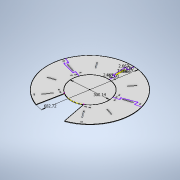
# Autodesk Inventor part: Ring Level 1 Full
Saved by Autodesk Inventor 2020 (Build 240168000, 168)
## iProperties
Created: 2020-03-10
Part Number: Ring Level 1 Full
Material: Generic
Document SubType Name: Sheet Metal
Designer: Daniel Wikman
Density: 1 g/cm^3
Sheet Metal Rule: Default_mm
Appearance: Default
Author: Daniel Wikman
Autodesk Inventor part; units mm, degrees
ref_plane "YZ Plane" through (0, 0, 0) normal (1, 0, 0) x (0, 1, 0)
ref_plane "XZ Plane" through (0, 0, 0) normal (0, 1, 0) x (-1, 0, 0)
sketch "Sketch1" plane through (0, 0, 0) normal (0, 1, 0) x (-1, 0, 0)
  circle A0 centre (0, 0) radius 341.36
  circle A1 centre (0, 0) radius 150.07
  dimension "d84" = 300.14
  dimension "d85" = 682.72
  constraints: 2 centre point, 1 coincident
  measures "d84" diameter of A1
  measures "d85" diameter of A0
extrude "Extrusion3" add sketch "Sketch1" along normal blind 6 contours A0 | A1
sketch "Sketch2" plane through (0, 6, 0) normal (0, 1, 0) x (1, 0, 0)
  circle A0 centre (0, 0) radius 245.715 construction
  line L0 (245.7148, 0.3131) -> (341.6521, -0.0088)
  line L1 (-0.6289, 279.0483) -> (-0.0524, 279.0483)
  line L2 (3.25, 279.0483) -> (3.25, 212.3817)
  line L3 (0.5377, 212.3817) -> (-0.051, 212.3817)
  line L4 (-3.25, 212.3817) -> (-3.25, 279.0483)
  arc A1 (-3.25, 212.3817) -> (-1.9167, 211.0483) centre (-1.9167, 212.3817) ccw
  arc A2 (1.9167, 211.0483) -> (3.25, 212.3817) centre (1.9167, 212.3817) ccw
  arc A3 (-1.9167, 280.3817) -> (-3.25, 279.0483) centre (-1.9167, 279.0483) ccw
  arc A4 (3.25, 279.0483) -> (1.9167, 280.3817) centre (1.9167, 279.0483) ccw
  line L5 (-1.9167, 280.3817) -> (1.9167, 280.3817)
  line L6 (-1.9167, 211.0483) -> (1.9167, 211.0483)
  line L7 (0, 0) -> (0, 212.3817)
  line L8 (0, 280.3817) -> (0, 341.36)
  line L9 (0, 211.0483) -> (0, 245.715) construction
  line L10 (0, 280.3817) -> (0, 245.715) construction
  arc A5 (-157.4948, 221.8428) -> (-159.3572, 222.1378) centre (-158.5735, 221.0591) ccw
  line L11 (-162.4585, 219.8846) -> (-159.3572, 222.1378)
  arc A6 (-162.4585, 219.8846) -> (-162.7534, 218.0222) centre (-161.6748, 218.8059) ccw
  line L12 (-160.9079, 221.0112) -> (-144.3647, 198.2416) construction
  line L13 (-160.633, 219.5628) -> (-160.1666, 219.9017)
  line L14 (-157.4948, 221.8428) -> (-125.976, 178.4609)
  line L15 (-131.2346, 174.6403) -> (-162.7534, 218.0222)
  line L16 (-127.8216, 175.4719) -> (-144.3647, 198.2416) construction
  line L17 (-128.1703, 176.8667) -> (-128.6466, 176.5206)
  arc A7 (-126.271, 176.5985) -> (-125.976, 178.4609) centre (-127.0547, 177.6772) ccw
  line L18 (-129.3722, 174.3453) -> (-126.271, 176.5985)
  arc A8 (-131.2346, 174.6403) -> (-129.3722, 174.3453) centre (-130.156, 175.424) ccw
  arc A9 (-259.6684, -81.8575) -> (-260.5244, -83.5376) centre (-259.2564, -83.1256) ccw
  line L19 (-259.3399, -87.1834) -> (-260.5244, -83.5376)
  arc A10 (-259.3399, -87.1834) -> (-257.6598, -88.0394) centre (-258.0718, -86.7713) ccw
  line L20 (-259.9321, -85.3605) -> (-233.1648, -76.6633) construction
  line L21 (-258.4697, -85.5466) -> (-258.6479, -84.9983)
  line L22 (-259.6684, -81.8575) -> (-208.6699, -65.2871)
  line L23 (-206.6613, -71.469) -> (-257.6598, -88.0394)
  line L24 (-206.3975, -67.966) -> (-233.1648, -76.6633) construction
  line L25 (-207.8317, -67.8666) -> (-207.6498, -68.4265)
  arc A11 (-206.9898, -66.1432) -> (-208.6699, -65.2871) centre (-208.2578, -66.5552) ccw
  line L26 (-205.8052, -69.7889) -> (-206.9898, -66.1432)
  arc A12 (-206.6613, -71.469) -> (-205.8052, -69.7889) centre (-207.0733, -70.2009) ccw
  arc A13 (258.6901, -87.4674) -> (260.3702, -86.6114) centre (259.1021, -86.1993) ccw
  line L27 (261.5548, -82.9657) -> (260.3702, -86.6114)
  arc A14 (261.5548, -82.9657) -> (260.6987, -81.2856) centre (260.2867, -82.5536) ccw
  line L28 (260.9625, -84.7885) -> (234.1951, -76.0913) construction
  line L29 (259.8887, -83.7783) -> (259.7106, -84.3266)
  line L30 (258.6901, -87.4674) -> (207.6916, -70.897)
  line L31 (209.7002, -64.7151) -> (260.6987, -81.2856)
  line L32 (207.4278, -67.394) -> (234.1951, -76.0913) construction
  line L33 (208.5297, -68.3175) -> (208.7116, -67.7576)
  arc A15 (206.8355, -69.2169) -> (207.6916, -70.897) centre (208.1036, -69.6289) ccw
  line L34 (208.0201, -65.5712) -> (206.8355, -69.2169)
  arc A16 (209.7002, -64.7151) -> (208.0201, -65.5712) centre (209.2882, -65.9832) ccw
  arc A17 (162.9147, 218.5186) -> (162.6198, 220.381) centre (161.836, 219.3023) ccw
  line L35 (159.5185, 222.6342) -> (162.6198, 220.381)
  arc A18 (159.5185, 222.6342) -> (157.6561, 222.3392) centre (158.7348, 221.5555) ccw
  line L36 (161.0691, 221.5076) -> (144.526, 198.7379) construction
  line L37 (159.7766, 220.7986) -> (160.243, 220.4597)
  line L38 (162.9147, 218.5186) -> (131.3959, 175.1367)
  line L39 (126.1373, 178.9573) -> (157.6561, 222.3392)
  line L40 (127.9829, 175.9683) -> (144.526, 198.7379) construction
  line L41 (129.2017, 176.7309) -> (128.7254, 177.0769)
  arc A19 (129.5335, 174.8417) -> (131.3959, 175.1367) centre (130.3172, 175.9204) ccw
  line L42 (126.4323, 177.0949) -> (129.5335, 174.8417)
  arc A20 (126.1373, 178.9573) -> (126.4323, 177.0949) centre (127.216, 178.1736) ccw
  line L43 (-265.5851, 85.6325) -> (-265.4069, 86.1808)
  line L44 (-267.2511, 84.8198) -> (-266.0665, 88.4656)
  line L45 (-201.3112, 63.3947) -> (-200.1266, 67.0404)
  arc A21 (-267.2511, 84.8198) -> (-266.395, 83.1397) centre (-265.983, 84.4078) ccw
  arc A22 (-264.3864, 89.3216) -> (-266.0665, 88.4656) centre (-264.7985, 88.0535) ccw
  line L46 (-266.6588, 86.6427) -> (-233.6889, 75.9301) construction
  line L47 (-202.9913, 62.5386) -> (-266.395, 83.1397)
  line L48 (-264.3864, 89.3216) -> (-200.9827, 68.7205)
  line L49 (-200.7189, 65.2175) -> (-233.6889, 75.9301) construction
  arc A23 (-202.9913, 62.5386) -> (-201.3112, 63.3947) centre (-202.5793, 63.8067) ccw
  arc A24 (-200.1266, 67.0404) -> (-200.9827, 68.7205) centre (-201.3947, 67.4524) ccw
  line L50 (-201.8208, 66.141) -> (-202.0027, 65.5811)
  line L51 (-163.5117, -226.1245) -> (-163.9781, -225.7857)
  line L52 (-163.2536, -227.9601) -> (-166.3548, -225.7069)
  line L53 (-122.5005, -171.8683) -> (-125.6017, -169.6151)
  arc A25 (-163.2536, -227.9601) -> (-161.3912, -227.6651) centre (-162.4699, -226.8814) ccw
  arc A26 (-166.6498, -223.8445) -> (-166.3548, -225.7069) centre (-165.5711, -224.6283) ccw
  line L54 (-164.8042, -226.8335) -> (-144.4277, -198.7876) construction
  line L55 (-122.2055, -173.7307) -> (-161.3912, -227.6651)
  line L56 (-166.6498, -223.8445) -> (-127.4641, -169.9101)
  line L57 (-124.0511, -170.7417) -> (-144.4277, -198.7876) construction
  arc A27 (-122.2055, -173.7307) -> (-122.5005, -171.8683) centre (-123.2842, -172.947) ccw
  arc A28 (-125.6017, -169.6151) -> (-127.4641, -169.9101) centre (-126.3854, -170.6938) ccw
  line L58 (-125.2699, -171.5043) -> (-124.7936, -171.8503)
  line L59 (164.5293, -225.3852) -> (164.0629, -225.724)
  line L60 (166.3548, -225.7069) -> (163.2536, -227.9601)
  line L61 (125.6017, -169.6151) -> (122.5005, -171.8683)
  arc A29 (166.3548, -225.7069) -> (166.6498, -223.8445) centre (165.5711, -224.6283) ccw
  arc A30 (161.3912, -227.6651) -> (163.2536, -227.9601) centre (162.4699, -226.8814) ccw
  line L62 (164.8042, -226.8335) -> (144.4277, -198.7876) construction
  line L63 (127.4641, -169.9101) -> (166.6498, -223.8445)
  line L64 (161.3912, -227.6651) -> (122.2055, -173.7307)
  line L65 (124.0511, -170.7417) -> (144.4277, -198.7876) construction
  arc A31 (127.4641, -169.9101) -> (125.6017, -169.6151) centre (126.3854, -170.6938) ccw
  arc A32 (122.5005, -171.8683) -> (122.2055, -173.7307) centre (123.2842, -172.947) ccw
  line L66 (124.3998, -172.1365) -> (124.8761, -171.7904)
  line L67 (265.1964, 86.8288) -> (265.3745, 86.2805)
  line L68 (266.0665, 88.4656) -> (267.2511, 84.8198)
  line L69 (200.1266, 67.0404) -> (201.3112, 63.3947)
  arc A33 (266.0665, 88.4656) -> (264.3864, 89.3216) centre (264.7985, 88.0535) ccw
  arc A34 (266.395, 83.1397) -> (267.2511, 84.8198) centre (265.983, 84.4078) ccw
  line L70 (266.6588, 86.6427) -> (233.6889, 75.9301) construction
  line L71 (200.9827, 68.7205) -> (264.3864, 89.3216)
  line L72 (266.395, 83.1397) -> (202.9913, 62.5386)
  line L73 (200.7189, 65.2175) -> (233.6889, 75.9301) construction
  arc A35 (200.9827, 68.7205) -> (200.1266, 67.0404) centre (201.3947, 67.4524) ccw
  arc A36 (201.3112, 63.3947) -> (202.9913, 62.5386) centre (202.5793, 63.8067) ccw
  line L74 (202.1531, 65.1181) -> (201.9712, 65.678)
  line L75 (236.8664, -101.279) -> (236.7913, -101.5102)
  point P0 (-128.6053, 176.5506)
  point P1 (-207.6656, -68.3781)
  point P2 (208.6959, -67.8061)
  point P3 (128.7666, 177.047)
  point P4 (-201.987, 65.6295)
  point P5 (-124.8348, -171.8204)
  point P6 (124.8348, -171.8204)
  point P7 (201.987, 65.6295)
  dimension "d21" = 6.5
  dimension "d23" = 66.6667
  dimension "d24" = 2.6667
  dimension "d25" = 2.6667
  dimension "d32" = 1.3333
  dimension "d33" = 1.3333
  dimension "d41" = 90
  dimension "d42" = 3.25
  dimension "d43" = 90
  dimension "d49" = 360
  dimension "d86" = 491.43
  dimension "d96" = 0.243
  constraints: 152 end point, 74 point on circle, 47 point on line, 37 centre point, 18 midpoint, 6 tangent, 2 collinear, 2 parallel, 2 vertical, 1 coincident, 1 horizontal, 1 perpendicular, 161 other
  measures "d21" distance between parallel lines of L2 L4
  measures "d23" distance between parallel lines of L1 L3
  measures "d24" diameter of A1
  measures "d25" diameter of A2
  measures "d32" radius of A3
  measures "d33" radius of A4
  measures "d41" angle of L6 L7
  measures "d42" distance between parallel lines of L7 L2
  measures "d43" angle of L5 L8
  measures "d86" diameter of A0
  measures "d96" distance of L75.start L75.end
extrude "Extrusion4" cut sketch "Sketch2" against normal through all
sketch "Sketch3" plane through (0, 6, 0) normal (0, 1, 0) x (1, 0, 0)
  arc A0 (-115.2299, -321.3234) -> (115.2355, -321.3214) centre (0, 0) ccw
  arc A1 (-77.7244, -128.3741) -> (77.7297, -128.3709) centre (0, 0) ccw
  line L0 (-122.1811, -173.696) -> (-161.3589, -227.6196)
  line L1 (-115.2299, -321.3234) -> (-77.7244, -128.3741)
  line L2 (0, 0) -> (0, -341.2918)
  line L3 (115.2355, -321.3214) -> (77.7297, -128.3709)
  line L4 (161.3912, -227.6651) -> (122.2055, -173.7307) projected
  dimension "d52" = 25
  dimension "d87" = 150.07
  dimension "d88" = 341.36
  dimension "d89" = 25
  dimension "d90" = 11
  dimension "d91" = 11
  constraints: 8 end point, 4 point on circle, 2 centre point, 1 coincident
  measures "d52" angle of L0 L1
  measures "d87" radius of A1
  measures "d88" radius of A0
  measures "d89" angle of L4 L3
  measures "d90" angle of L3 L2
  measures "d91" angle of L1 L2
extrude "Extrusion5" cut sketch "Sketch3" against normal blind 10
sketch "Sketch5" plane through (0, 6, 0) normal (0, 1, 0) x (1, 0, 0)
  line L0 (3.25, 279.0483) -> (3.25, 212.3817) projected
  line L1 (5.5862, 197.9634) -> (-6.155, 194.8174)
  line L2 (-11.2263, 301.7146) -> (10.5847, 293.3421)
  line L3 (6.5657, 149.9554) -> (8.9394, 195.248)
  line L4 (14.2034, 295.6921) -> (16.5771, 340.9846)
  arc A0 (10.5847, 293.3421) -> (14.2034, 295.6921) centre (11.5404, 295.8316) ccw
  arc A1 (8.9394, 195.248) -> (5.5862, 197.9634) centre (6.2763, 195.3876) ccw
  arc A2 (-11.2263, 301.7146) -> (-14.8449, 299.0854) centre (-12.1819, 299.225) ccw
  line L5 (-3.25, 212.3817) -> (-3.25, 279.0483) projected
  line L6 (-14.8449, 299.0854) -> (-9.5081, 197.2536)
  arc A3 (-9.5081, 197.2536) -> (-6.155, 194.8174) centre (-6.8451, 197.3932) ccw
  line L7 (-1.9167, 211.0483) -> (1.9167, 211.0483) projected
  line L8 (1.9167, 280.3817) -> (-1.9167, 280.3817) projected
  arc A4 (115.2355, -321.3214) -> (-115.2299, -321.3234) centre (0, 0) ccw
  line L9 (16.5771, 340.9846) -> (16.5774, 340.9903)
  arc A5 (-190.5375, 51.9119) -> (-187.1843, 54.3482) centre (-189.8473, 54.4877) ccw
  line L10 (-186.5481, 66.4868) -> (-187.1843, 54.3482)
  arc A6 (-182.9295, 68.8368) -> (-186.5481, 66.4868) centre (-183.8851, 66.3472) ccw
  arc A7 (-275.714, 100.7144) -> (-276.8308, 104.8821) centre (-277.7864, 102.3926) ccw
  line L11 (-289.0345, 78.3041) -> (-190.5375, 51.9119)
  arc A8 (-290.4167, 82.5581) -> (-289.0345, 78.3041) centre (-288.3443, 80.8799) ccw
  line L12 (-290.4167, 82.5581) -> (-275.714, 100.7144)
  line L13 (-276.8308, 104.8821) -> (-319.1731, 121.1358)
  line L14 (-140.5872, 52.5831) -> (-182.9295, 68.8368)
  line L15 (-319.1731, 121.1358) -> (-319.1784, 121.1378)
  arc A9 (184.6611, 69.9975) -> (183.3803, 66.0556) centre (185.6168, 67.508) ccw
  line L16 (190.0006, 55.8613) -> (183.3803, 66.0556)
  arc A10 (188.4543, 51.8331) -> (190.0006, 55.8613) centre (187.7641, 54.4089) ccw
  arc A11 (282.2558, 80.581) -> (285.609, 77.8656) centre (284.9188, 80.4414) ccw
  line L17 (279.8598, 106.5409) -> (184.6611, 69.9975)
  arc A12 (283.4785, 103.9117) -> (279.8598, 106.5409) centre (280.8155, 104.0513) ccw
  line L18 (283.4785, 103.9117) -> (282.2558, 80.581)
  line L19 (285.609, 77.8656) -> (329.4183, 89.6043)
  line L20 (144.645, 40.0945) -> (188.4543, 51.8331)
  line L21 (329.4183, 89.6043) -> (329.4238, 89.6058)
  circle A13 centre (0, 0) radius 150.07
  line L22 (-140.5872, 52.5831) -> (-140.5479, 52.568)
  line L23 (144.645, 40.0945) -> (144.5122, 40.0589)
  line L24 (6.5657, 149.9554) -> (6.5621, 149.8874)
  arc A14 (-77.7244, -128.3741) -> (77.7297, -128.3709) centre (0, 0) ccw projected
  arc A15 (115.2355, -321.3214) -> (-115.2299, -321.3234) centre (0, 0) ccw projected
  line L25 (77.7297, -128.3709) -> (115.2355, -321.3214)
  line L26 (-77.7244, -128.3741) -> (-115.2299, -321.3234)
  point P0 (-77.7399, -128.3998)
  point P1 (77.7399, -128.3998)
  point P2 (-319.1475, 121.126)
  point P3 (-140.56, 52.5727)
  point P4 (6.5642, 149.9264)
  point P5 (16.5757, 340.9573)
  point P6 (329.3918, 89.5972)
  point P7 (144.6169, 40.0869)
  dimension "d63" = 2.6667
  dimension "d64" = 3
  dimension "d66" = 3
  dimension "d67" = 2.6667
  dimension "d68" = 2.6667
  dimension "d70" = 72
  dimension "d71" = 72
  dimension "d94" = 300.14
  dimension "d95" = 682.72
  constraints: 46 end point, 26 point on circle, 14 centre point, 8 tangent, 2 collinear, 1 coincident, 1 equal radius
  measures "d63" radius of A0
  measures "d64" angle of L0 L4
  measures "d66" angle of L5 L6
  measures "d67" radius of A2
  measures "d68" radius of A3
  measures "d70" angle of L3 L1
  measures "d71" angle of L4 L2
  measures "d94" diameter of A13
  measures "d95" diameter of A4
sketch "Sketch6" plane through (0, 6, 0) normal (0, 1, 0) x (1, 0, 0)
  line L0 (188.7727, -264.2184) -> (198.4809, -257.165)
  line L1 (194.6603, -251.9064) -> (184.9521, -258.9598)
  line L2 (161.3912, -227.6651) -> (122.2055, -173.7307) projected
  line L3 (166.3548, -225.7069) -> (163.2536, -227.9601) projected
  arc A0 (195.5915, -252.0539) -> (194.6603, -251.9064) centre (195.0522, -252.4457) ccw
  arc A1 (198.4809, -257.165) -> (198.6284, -256.2338) centre (198.0891, -256.6256) ccw
  arc A2 (187.8415, -264.0709) -> (188.7727, -264.2184) centre (188.3809, -263.6791) ccw
  arc A3 (184.9521, -258.9598) -> (184.8046, -259.891) centre (185.344, -259.4991) ccw
  line L4 (184.8046, -259.891) -> (187.8415, -264.0709)
  line L5 (198.6284, -256.2338) -> (195.5915, -252.0539)
  line L6 (122.2055, -173.7307) -> (161.3912, -227.6651) projected
  line L7 (141.7983, -200.6979) -> (147.057, -196.8773)
  line L8 (166.6498, -223.8445) -> (127.4641, -169.9101) projected
  line L9 (95.9027, -136.3937) -> (105.6109, -129.3403)
  line L10 (109.4315, -134.5989) -> (99.7233, -141.6523)
  arc A4 (109.4315, -134.5989) -> (109.579, -133.6677) centre (109.0396, -134.0596) ccw
  arc A5 (106.5421, -129.4878) -> (105.6109, -129.3403) centre (106.0027, -129.8796) ccw
  arc A6 (95.9027, -136.3937) -> (95.7552, -137.3249) centre (96.2945, -136.9331) ccw
  arc A7 (98.7921, -141.5048) -> (99.7233, -141.6523) centre (99.3314, -141.113) ccw
  line L11 (98.7921, -141.5048) -> (95.7552, -137.3249)
  line L12 (106.5421, -129.4878) -> (109.579, -133.6677)
  point P0 (0, 0)
  dimension "d104" = 6.5
  dimension "d105" = 12
  dimension "d108" = 1.3333
  dimension "d109" = 1.3333
  dimension "d110" = 1.3333
  dimension "d111" = 1.3333
  dimension "d112" = 0
  dimension "d149" = 145
  dimension "d150" = 90
  dimension "d151" = 90
  dimension "d152" = 90
  dimension "d153" = 90
  constraints: 18 end point, 16 point on circle, 12 symmetric about line, 8 centre point, 8 tangent, 2 midpoint, 4 other
  measures "d104" distance of L1.end L0.start
  measures "d105" distance of L0.start L0.end
  measures "d108" diameter of A0
  measures "d109" diameter of A1
  measures "d110" diameter of A2
  measures "d111" diameter of A3
  measures "d112" distance between parallel lines of L2 L4
  measures "d149" diameter of L1 L7
  measures "d150" angle of L5 L1
  measures "d151" angle of L0 L5
  measures "d152" angle of L4 L0
  measures "d153" angle of L1 L4
extrude "Extrusion7" cut sketch "Sketch6" against normal through all
sketch "Sketch7" plane through (0, 6, 0) normal (0, 1, 0) x (1, 0, 0)
  line L0 (119.5964, -125.4786) -> (127.6865, -119.6008)
  line L1 (106.4838, -136.3528) -> (96.7756, -143.4062)
  line L2 (128.6177, -119.7483) -> (131.6546, -123.9282)
  line L3 (131.5071, -124.8594) -> (123.417, -130.7373)
  line L4 (122.4858, -130.5898) -> (119.4489, -126.4098)
  line L5 (103.5944, -131.2417) -> (106.6313, -135.4216)
  arc A0 (119.5964, -125.4786) -> (119.4489, -126.4098) centre (119.9882, -126.018) ccw
  arc A1 (122.4858, -130.5898) -> (123.417, -130.7373) centre (123.0251, -130.1979) ccw
  arc A2 (128.6177, -119.7483) -> (127.6865, -119.6008) centre (128.0784, -120.1401) ccw
  arc A3 (131.5071, -124.8594) -> (131.6546, -123.9282) centre (131.1153, -124.3201) ccw
  line L6 (173.6068, 21.7165) -> (170.5167, 31.227)
  line L7 (170.9447, 32.0671) -> (175.8585, 33.6637)
  line L8 (176.6985, 33.2357) -> (179.7887, 23.7251)
  line L9 (179.3607, 22.885) -> (174.4469, 21.2885)
  arc A4 (173.6068, 21.7165) -> (174.4469, 21.2885) centre (174.2409, 21.9225) ccw
  arc A5 (179.3607, 22.885) -> (179.7887, 23.7251) centre (179.1547, 23.5191) ccw
  arc A6 (170.9447, 32.0671) -> (170.5167, 31.227) centre (171.1507, 31.4331) ccw
  arc A7 (176.6985, 33.2357) -> (175.8585, 33.6637) centre (176.0645, 33.0296) ccw
  line L10 (188.4543, 51.8331) -> (144.6169, 40.0869) projected
  line L11 (201.3112, 63.3947) -> (200.1266, 67.0404) projected
  line L12 (179.8921, 12.7927) -> (180.0981, 12.1586)
  line L13 (183.5904, 29.3861) -> (183.8471, 29.4696)
  point P0 (0, 0)
  dimension "d116" = 1.3333
  dimension "d117" = 1.3333
  dimension "d119" = 1.3333
  dimension "d120" = 1.3333
  dimension "d121" = 6.5
  dimension "d122" = 10
  dimension "d126" = 1.09
  dimension "d127" = 16.3333
  dimension "d128" = 1.3333
  dimension "d129" = 1.3333
  dimension "d130" = 1.3333
  dimension "d131" = 1.3333
  dimension "d132" = 6.5
  dimension "d133" = 10
  dimension "d135" = 3
  dimension "d140" = 0.6667
  dimension "d148" = 0.27
  constraints: 24 end point, 16 point on circle, 8 centre point
  measures "d116" diameter of A0
  measures "d117" diameter of A1
  measures "d119" diameter of A2
  measures "d120" diameter of A3
  measures "d121" distance between parallel lines of L3 L0
  measures "d122" distance of L3.start L3.end
  measures "d126" distance between parallel lines of L1 L0
  measures "d127" distance from line of L5 L0.start
  measures "d128" diameter of A4
  measures "d129" diameter of A5
  measures "d130" diameter of A6
  measures "d131" diameter of A7
  measures "d132" distance between parallel lines of L8 L6
  measures "d133" distance of L8.start L8.end
  measures "d135" angle of L10 L7
  measures "d140" distance of L12.start L12.end
  measures "d148" distance of L13.start L13.end
extrude "Extrusion8" cut sketch "Sketch7" against normal through all contours L0 A2 L2 A3 L3 A1 L4 A0
extrude "Extrusion9" cut sketch "Sketch7" against normal through all contours L6 A6 L7 A7 L8 A5 L9 A4
ref_plane "Work Plane1" through (265.3907, 0, -86.2307) normal (0.309, 0, 0.9511) x (0.9511, 0, -0.309)
mirror "Mirror2" about plane through (265.3907, 0, -86.2307) normal (0.309, 0, 0.9511) of "Extrusion9"
mirror "Mirror1" about plane through (0, 0, 0) normal (1, 0, 0) of "Extrusion8", "Extrusion9", "Mirror2"
pattern_circular "Circular Pattern1" count 2 over 72 about axis through (0, -10, 0) along (0, 1, 0) of "Extrusion9", "Mirror2"
pattern_circular "Circular Pattern2" count 2 over 72 about axis through (0, -10, 0) along (0, 1, 0) of "Extrusion7"
pattern_circular "Circular Pattern3" count 2 over 144 about axis through (0, -10, 0) along (0, 1, 0) of "Extrusion7"
mirror "Mirror3" about plane through (0, 0, 0) normal (1, 0, 0) of "Extrusion7"
pattern_circular "Circular Pattern4" count 2 over 144 about axis through (0, -10, 0) along (0, -1, 0) of "Extrusion7"
equation "\"BendRadius\" = Thickness"
equation "\"BendReliefWidth\" = Thickness"
equation "\"BendReliefDepth\" = 0.5 * Thickness"
equation "\"CornerReliefSize\" = 4 * Thickness"
equation "\"MinimumRemnant\" = 2 * Thickness"
equation "\"TransitionRadius\" = BendRadius"
equation "\"JacobiRadiusSize\" = BendRadius"
equation "\"GapSize\" = Thickness"
equation "\"Thickness\" = 0.5"
body "Solid3"
